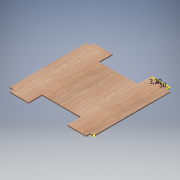
# Autodesk Inventor part: middle plate
Saved by Autodesk Inventor 2018.1 (Build 221171000, 171)
## iProperties
Created: 2017-11-11
Part Number: middle plate
Material: Birke
Document SubType Name: Modeling
Designer: Till
Density: 0.512 g/cm^3
Appearance: Birke - natur - mittlerer Glanz
Author: Till
Autodesk Inventor part; units mm, degrees
ref_plane "YZ Plane" through (0, 0, 0) normal (1, 0, 0) x (0, 1, 0)
ref_plane "XZ Plane" through (0, 0, 0) normal (0, 1, 0) x (-1, 0, 0)
ref_plane "XY Plane" through (0, 0, 0) normal (0, 0, 1) x (1, 0, 0)
sketch "Skizze1" plane through (0, 0, 0) normal (0, 0, 1) x (1, 0, 0)
  line L0 (0, 0) -> (0, 395)
  line L1 (0, 395) -> (-20, 395)
  line L2 (-20, 395) -> (-20, 415)
  line L3 (-20, 415) -> (-117.5, 415)
  line L4 (-117.5, 415) -> (-117.5, 345)
  line L5 (-117.5, 345) -> (-317.5, 345)
  line L6 (-317.5, 345) -> (-317.5, 415)
  line L7 (-317.5, 415) -> (-415, 415)
  line L8 (-415, 415) -> (-415, 395)
  line L9 (-415, 395) -> (-435, 395)
  line L10 (-435, 395) -> (-435, 0)
  line L11 (-435, 0) -> (-415, 0)
  line L12 (-415, 0) -> (-415, -20)
  line L13 (-415, 0) -> (-395, 0) construction
  line L14 (-415, -20) -> (-317.5, -20)
  line L15 (-317.5, -20) -> (-317.5, 50)
  line L16 (-317.5, 50) -> (-117.5, 50)
  line L17 (-117.5, 50) -> (-117.5, -20)
  line L18 (-117.5, -20) -> (-20, -20)
  line L19 (-20, -20) -> (-20, 0)
  line L20 (-20, 0) -> (0, 0)
  dimension "d0" = 395
  dimension "d1" = 20
  dimension "d2" = 20
  dimension "d3" = 97.5
  dimension "d4" = 90
  dimension "d5" = 70
  dimension "d6" = 90
  dimension "d7" = 200
  dimension "d8" = 70
  dimension "d9" = 90
  dimension "d10" = 97.5
  dimension "d11" = 20
  dimension "d12" = 90
  dimension "d13" = 20
  dimension "d14" = 90
  dimension "d15" = 395
  dimension "d16" = 90
  dimension "d17" = 20
  dimension "d18" = 20
  dimension "d19" = 90
  dimension "d20" = 70
  dimension "d21" = 90
  constraints: 42 end point, 16 perpendicular, 4 point on line, 2 vertical, 1 horizontal
  measures "d0" distance of L0.start L0.end
  measures "d1" distance of L0.end L1.end
  measures "d2" distance of L1.end L2.end
  measures "d3" distance of L2.end L3.end
  measures "d4" angle of L3 L2
  measures "d5" distance of L3.end L4.end
  measures "d6" angle of L4 L3
  measures "d7" distance of L4.end L5.end
  measures "d8" distance of L5.end L6.end
  measures "d9" angle of L5 L6
  measures "d10" distance of L6.end L7.end
  measures "d11" distance of L7.end L8.end
  measures "d12" angle of L8 L7
  measures "d13" distance of L8.end L9.end
  measures "d14" angle of L8 L9
  measures "d15" distance of L9.end L10.end
  measures "d16" angle of L10 L9
  measures "d17" distance of L10.end L11.end
  measures "d18" distance of L11.end L12.end
  measures "d19" angle of L12 L13
  measures "d20" distance of L14.end L15.end
  measures "d21" angle of L15 L14
extrude "Extrusion1" add sketch "Skizze1" along normal blind 6
chamfer "Fase1" distance 0.5 angle 45 40 edges at (0, 197.5, 6) (-10, 0, 6) (-20, -10, 6) (-68.75, -20, 6) (-117.5, 15, 6) (-217.5, 50, 6) (-317.5, 15, 6) (-366.25, -20, 6) (-415, -10, 6) (-425, 0, 6) (-435, 197.5, 6) (-425, 395, 6) (-366.25, 415, 6) (-415, 405, 6) (-317.5, 380, 6) (-217.5, 345, 6) (-117.5, 380, 6) (-68.75, 415, 6) (-20, 405, 6) (-10, 395, 6) (-425, 0, 0) (-415, -10, 0) (-435, 197.5, 0) (-366.25, -20, 0) (-217.5, 50, 0) (-317.5, 15, 0) (-117.5, 15, 0) (-68.75, -20, 0) (-20, -10, 0) (-10, 0, 0) (0, 197.5, 0) (-10, 395, 0) (-20, 405, 0) (-68.75, 415, 0) (-117.5, 380, 0) (-217.5, 345, 0) (-317.5, 380, 0) (-425, 395, 0) (-415, 405, 0) (-366.25, 415, 0)
sketch "Skizze2" plane through (0, 0, 6) normal (0, 0, 1) x (1, 0, 0)
  circle A0 centre (-70.5, 407) radius 1.6
  line L0 (-117, 414.5) -> (-20.5, 414.5) projected
  line L1 (-20.5, 414.5) -> (-20.5, 394.5) projected
  circle A1 centre (-370.5, 407) radius 1.6
  circle A2 centre (-70.5, -13) radius 1.6
  circle A3 centre (-370.5, -13) radius 1.6
  point P0 (0, 0)
  dimension "d27" = 3.2
  dimension "d28" = 7.5
  dimension "d29" = 50
  dimension "d32" = 300
  dimension "d35" = 420
  constraints: 4 centre point, 1 horizontal, 1 vertical, 6 other
  measures "d27" diameter of A0
  measures "d28" distance from line of L0 A0.centre
  measures "d29" distance from line of A0.centre L1
  measures "d32" distance of A0.centre A1.centre
  measures "d35" distance of A0.centre A2.centre
extrude "Extrusion2" cut sketch "Skizze2" against normal through all
